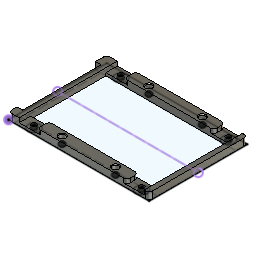
Amiga 600 1200 HDD adapter frame (Autodesk Fusion 360 design; units mm, degrees)
Autodesk Fusion 360 part; units mm, degrees
note: some values were not read from the file. Set by a fixed rule: which sketch regions a step uses.
sketch "Drive size" plane through (0, 0, 0) normal (0, 0, 1) x (1, 0, 0)
  line L0 (0, 0) -> (100, 0)
  line L1 (100, 0) -> (100, 69.85)
  line L2 (100, 69.85) -> (0, 69.85)
  line L3 (0, 69.85) -> (0, 0)
  line L4 (0, 34.925) -> (100, 34.925) construction
  line L5 (4, 69.85) -> (4, 0) construction
  line L6 (0, 61.85) -> (100, 61.85) construction
  line L7 (0, 6) -> (100, 6) construction
  dimension "d1" = 100
  dimension "d2" = 69.85
  dimension "d19" = 4
  dimension "d20" = 8
  dimension "d21" = 6
  constraint horizontal L0
  constraint vertical L1
  constraint horizontal L2
  constraint vertical L3
  constraint coincident L0.start L3.end
  constraint midpoint L3 L4.start
  constraint midpoint L1 L4.end
  constraint coincident L2 L5.start
  constraint coincident L0 L5.end
  constraint perpendicular L0 L5
  constraint coincident L3 L6.start
  constraint coincident L1 L6.end
  constraint perpendicular L1 L6
  constraint coincident L3 L7.start
  constraint coincident L1 L7.end
  constraint perpendicular L1 L7
  measures "d1" distance of L1.end L2.end
  measures "d2" distance of L0.end L1.end
  measures "d19" distance of L0.start L5.end
  measures "d20" distance of L2.end L6.start
  measures "d21" distance of L0.start L7.start
sketch "Hole positions" plane through (0, 0, 0) normal (0, 0, 1) x (1, 0, 0)
  circle A0 centre (34, 4.07) radius 2.125
  circle A1 centre (72, 4.07) radius 2.125
  circle A2 centre (14, 4.07) radius 1.75
  circle A3 centre (90.6, 4.07) radius 1.75
  circle A4 centre (14, 4.07) radius 4.07
  circle A5 centre (90.6, 4.07) radius 4.07
  line L0 (0, 34.925) -> (100, 34.925)
  circle A6 centre (14, 65.78) radius 4.07
  circle A7 centre (14, 65.78) radius 1.75
  circle A8 centre (34, 65.78) radius 2.125
  circle A9 centre (72, 65.78) radius 2.125
  circle A10 centre (90.6, 65.78) radius 4.07
  circle A11 centre (90.6, 65.78) radius 1.75
  point P0 (34, 4.07)
  point P1 (72, 4.07)
  point P2 (34, 65.78)
  point P3 (72, 65.78)
  dimension "d5" = 34
  dimension "d7" = 4.07
  dimension "d8" = 14
  dimension "d9" = 90.6
  dimension "d10" = 72
  dimension "d11" = 3.5
  dimension "d12" = 4.25
  dimension "d13" = 4.25
  dimension "d14" = 3.5
  dimension "d17" = 8.14
  dimension "d18" = 8.14
  constraint horizontal P0 A1.centre
  constraint horizontal P0 A3.centre
  constraint horizontal P0 A2.centre
  constraint concentric A2 A4
  constraint concentric A3 A5
  constraint symmetric A0 L0 A8
  constraint symmetric A1 L0 A9
  constraint symmetric A2 L0 A7
  constraint symmetric A3 L0 A11
  constraint symmetric A4 L0 A6
  constraint symmetric A5 L0 A10
  constraint coincident P0 A0.centre
  constraint coincident P1 A1.centre
  constraint coincident P2 A8.centre
  constraint coincident P3 A9.centre
  measures "d5" horizontal distance of P0 origin
  measures "d7" vertical distance of P0 origin
  measures "d8" horizontal distance of origin A2.centre
  measures "d9" horizontal distance of origin A3.centre
  measures "d10" horizontal distance of P1 origin
  measures "d11" diameter of A2
  measures "d12" diameter of A0
  measures "d13" diameter of A1
  measures "d14" diameter of A3
  measures "d17" diameter of A4
  measures "d18" diameter of A5
sketch "Sketch1" plane through (0, 0, 0) normal (0, 0, 1) x (1, 0, 0) in component "Adapter frame"
  line L0 (0, 0) -> (100, 0) construction
  line L1 (100, 0) -> (100, 69.85) construction
  line L2 (100, 69.85) -> (0, 69.85) construction
  line L3 (0, 69.85) -> (0, 0) construction
  circle A0 centre (90.6, 65.78) radius 4.07 construction
  circle A1 centre (90.6, 65.78) radius 1.75
  circle A2 centre (72, 65.78) radius 2.125
  circle A3 centre (34, 65.78) radius 2.125
  circle A4 centre (14, 65.78) radius 4.07 construction
  circle A5 centre (14, 65.78) radius 1.75
  line L4 (4, 69.85) -> (4, 0) construction
  line L5 (0, 34.925) -> (100, 34.925) construction
  circle A6 centre (14, 4.07) radius 4.07 construction
  circle A7 centre (14, 4.07) radius 1.75
  circle A8 centre (34, 4.07) radius 2.125
  circle A9 centre (90.6, 4.07) radius 4.07 construction
  circle A10 centre (90.6, 4.07) radius 1.75
  line L6 (0, 61.85) -> (100, 61.85) construction
  line L7 (9.93, 69.85) -> (9.93, 0)
  line L8 (18.07, 69.85) -> (18.07, 0)
  line L9 (86.53, 69.85) -> (86.53, 0)
  line L10 (94.67, 69.85) -> (94.67, 0)
  circle A11 centre (72, 4.07) radius 2.125
  line L11 (0, 69.85) -> (0, 61.85)
  line L12 (4, 61.85) -> (0, 61.85)
  line L13 (4, 61.85) -> (4, 6)
  line L14 (4, 6) -> (0, 6)
  line L15 (0, 6) -> (0, 0)
  line L16 (0, 0) -> (100, 0)
  line L17 (100, 0) -> (100, 69.85)
  line L18 (100, 69.85) -> (0, 69.85)
  line L19 (4, 8.14) -> (100, 8.14)
  line L20 (100, 61.71) -> (4, 61.71)
  line L21 (7.5, 69.85) -> (7.5, 0)
  line L22 (96.5, 69.85) -> (96.5, 0)
  line L23 (62, 0) -> (62, 69.85)
  line L24 (44, 0) -> (44, 69.85)
  line L25 (4, 6) -> (7.5, 6)
  line L26 (20.5, 0) -> (20.5, 69.85)
  line L27 (84.1, 0) -> (84.1, 69.85)
  point P0 (34, 65.78)
  dimension "d22" = 3.5
  dimension "d23" = 3.5
  dimension "d38" = 8.14
  dimension "d70" = 20
  dimension "d71" = 18.6
  dimension "d72" = 14.53
  dimension "d73" = 15.93
  dimension "d74" = 10
  dimension "d75" = 10
  dimension "d94" = 6
  dimension "d112" = 2.43
  dimension "d113" = 2.43
  dimension "d114" = 1.83
  dimension "d115" = 2.43
  constraint coincident L2 L7.start
  constraint coincident L0 L7.end
  constraint perpendicular L0 L7
  constraint coincident L2 L8.start
  constraint coincident L0 L8.end
  constraint perpendicular L0 L8
  constraint coincident L2 L9.start
  constraint coincident L0 L9.end
  constraint perpendicular L0 L9
  constraint coincident L2 L10.start
  constraint coincident L0 L10.end
  constraint perpendicular L0 L10
  constraint tangent A0 L9
  constraint tangent A0 L10
  constraint tangent A4 L8
  constraint tangent A4 L7
  constraint coincident L2.end L3.start
  constraint coincident L6.start L11.end
  constraint coincident L4 L12.start
  constraint coincident L6 L12.start
  constraint coincident L4 L13.end
  constraint coincident L0.start L3.end
  constraint coincident L0.end L1.start
  constraint perpendicular L2 L17
  constraint coincident L1.end L2.start
  constraint coincident L13 L19.start
  constraint coincident L1 L19.end
  constraint perpendicular L1 L19
  constraint tangent A9 L19
  constraint coincident L1 L20.start
  constraint coincident L4 L20.end
  constraint tangent A0 L20
  constraint coincident L2 L21.start
  constraint coincident L16 L21.end
  constraint perpendicular L16 L21
  constraint coincident L2 L22.start
  constraint coincident L0 L22.end
  constraint perpendicular L0 L22
  constraint coincident L0 L23.start
  constraint coincident L2 L23.end
  constraint perpendicular L2 L23
  constraint coincident L0 L24.start
  constraint coincident L2 L24.end
  constraint perpendicular L2 L24
  constraint coincident L21 L25.end
  constraint perpendicular L21 L25
  constraint horizontal L14.end L25.end
  constraint coincident L16 L26.start
  constraint coincident L18 L26.end
  constraint perpendicular L18 L26
  constraint coincident L16 L27.start
  constraint coincident L2 L27.end
  constraint perpendicular L2 L27
  measures "d22" horizontal distance of L13.end L21.end
  measures "d23" distance of L0.end L22.end
  measures "d38" diameter of A0
  measures "d70" distance of A6.centre A8.centre
  measures "d71" distance of A9.centre A11.centre
  measures "d72" horizontal distance of L9.end A11.centre
  measures "d73" horizontal distance of A8.centre L8.end
  measures "d74" horizontal distance of A11.centre L23.start
  measures "d75" horizontal distance of A8.centre L24.start
  measures "d94" distance of L14.end L0.start
  measures "d112" distance of L7.end L21.end
  measures "d113" distance of L8.end L26.start
  measures "d114" distance of L10.end L22.end
  measures "d115" distance of L9.end L27.start
extrude "Extrude20" add sketch "Sketch1" along normal blind 5 contours A2 | A3 | A8 | L7 L8 L18 L20 | L7 L18 L20 L21 | L8 L18 L20 L26 | L11 L12 L13 L18 L20 L21 | L7 L8 L16 L19 | L7 L16 L19 L21 | L13 L19 L20 L21 | L18 L20 L24 L26 | L13 L19 L21 L25 | L8 L16 L19 L26 | L18 L20 L23 L24 | L14 L15 L16 L21 L25 | L16 L19 L24 L26 | L18 L20 L23 L27 | L16 L19 L23 L24 | L9 L18 L20 L27 | L16 L19 L23 L27 | L9 L10 L18 L20 | L9 L16 L19 L27 | L10 L18 L20 L22 | L9 L10 L16 L19 | L17 L18 L20 L22 | L10 L16 L19 L22 | L17 L19 L20 L22 | L16 L17 L19 L22 | A11 in component "Adapter frame"
extrude "Extrude21" cut sketch "Sketch1" along normal up to surface (5 mm away) contours A2 | A3 | A8 | A11 in component "Adapter frame"
extrude "Extrude22" add sketch "Sketch1" along normal blind 1 contours A2 | A3 | A8 | A11 in component "Adapter frame"
ref_plane "WorkPlane1" through (0, 0, 4.5) normal (0, 0, 1) x (1, 0, 0) in component "Adapter frame"
sketch "Sketch5" plane through (0, 0, 5) normal (0, 0, 1) x (-1, 0, 0) in component "Adapter frame"
  circle A0 centre (-72, -65.78) radius 2.125
  circle A1 centre (-72, -4.07) radius 2.125
  circle A2 centre (-34, -65.78) radius 2.125
  circle A3 centre (-34, -4.07) radius 2.125
  circle A4 centre (-90.6, -65.78) radius 1.75
  circle A5 centre (-14, -65.78) radius 1.75
  circle A6 centre (-14, -4.07) radius 1.75
  line L0 (-7.5, -61.71) -> (-96.5, -61.71)
  line L1 (-96.5, -61.71) -> (-96.5, -8.14)
  line L2 (-96.5, -8.14) -> (-7.5, -8.14)
  line L3 (-7.5, -8.14) -> (-7.5, -61.71)
  circle A7 centre (-90.6, -4.07) radius 1.75
  line L4 (-4, -61.85) -> (-4, -6)
  line L5 (-4, -6) -> (0, -6)
  line L6 (0, -6) -> (0, 0)
  line L7 (0, 0) -> (-100, 0)
  line L8 (-100, 0) -> (-100, -69.85)
  line L9 (-100, -69.85) -> (0, -69.85)
  line L10 (0, -69.85) -> (0, -61.85)
  line L11 (0, -61.85) -> (-4, -61.85)
  line L12 (-7.5, -69.85) -> (-7.5, 0)
  line L13 (-20.5, 0) -> (-20.5, -69.85)
  line L14 (-100, -69.85) -> (0, -69.85)
  line L15 (-100, -61.71) -> (-4, -61.71)
  line L16 (-84.1, 0) -> (-84.1, -69.85)
  line L17 (-96.5, -69.85) -> (-96.5, 0)
  line L18 (0, 0) -> (-100, 0)
  line L19 (-4, -8.14) -> (-100, -8.14)
extrude "Extrude24" cut sketch "Sketch5" against normal blind 3 contours L0 L9 L12 L13 L14 L15 | L2 L7 L12 L13 L18 L19 | L0 L9 L14 L15 L16 L17 | L2 L7 L16 L17 L18 L19 in component "Adapter frame"
fillet "Fillet5" radius 2.5 12 edges at (0, 69.85, 2.5) (100, 69.85, 2.5) (100, 0, 2.5) (84.1, 69.85, 3.5) (84.1, 61.71, 3.5) (84.1, 8.14, 3.5) (84.1, 0, 3.5) (20.5, 69.85, 3.5) (20.5, 8.14, 3.5) (20.5, 61.71, 3.5) (0, 0, 2.5) (20.5, 0, 3.5) in component "Adapter frame"
chamfer "Chamfer1" distance 0.5 angle 45 4 edges at (32.0188, 66.5484, 5) (70.0188, 4.8384, 5) (32.0188, 4.8384, 5) (70.0188, 66.5484, 5) in component "Adapter frame"
component "Adapter frame" placed x (1, 0, 0) y (0, 1, 0) z (0, 0, 1) at (0, 0, 0)
equation "d13 = d12"
equation "d14 = d11"
equation "d15 = d7 * 2"
equation "d17 = d7 * 2"
equation "d18 = d17"
equation "d23 = d22"
equation "d113 = d112"
equation "d115 = d113"
named bodies: "A1200 HDD adapter frame"
